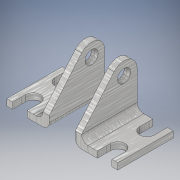
# Autodesk Inventor part: CylinderPivotMount_1.0625
Saved by Autodesk Inventor 2017 (Build 210142000, 142)
## iProperties
Created: 2017-01-24
Part Number: CylinderPivotMount_1.0625
Material: Steel
Document SubType Name: Modeling
Designer: Beezy
Density: 7.85 g/cm^3
Appearance: Polished Brushed
Author: Beezy
Autodesk Inventor part; units mm, degrees
ref_plane "YZ Plane" through (0, 0, 0) normal (1, 0, 0) x (0, 1, 0)
ref_plane "XZ Plane" through (0, 0, 0) normal (0, 1, 0) x (-1, 0, 0)
ref_plane "XY Plane" through (0, 0, 0) normal (0, 0, 1) x (1, 0, 0)
sketch "Sketch1" plane through (0, 0, 0) normal (0, 0, 1) x (1, 0, 0)
  line L0 (0, 0) -> (0, 44.7575) construction
  line L1 (-26.924, 0) -> (-26.924, 3.048)
  line L2 (-26.924, 3.048) -> (-12.573, 3.048)
  line L3 (-9.398, 6.223) -> (-9.398, 26.924)
  line L4 (-9.398, 26.924) -> (-6.35, 26.924)
  line L5 (-6.35, 26.924) -> (-6.35, 3.175)
  line L6 (-9.525, 0) -> (-26.924, 0)
  arc A0 (-9.525, 0) -> (-6.35, 3.175) centre (-9.525, 3.175) ccw
  arc A1 (-12.573, 3.048) -> (-9.398, 6.223) centre (-12.573, 6.223) ccw
  line L7 (26.924, 0) -> (26.924, 3.048)
  line L8 (26.924, 3.048) -> (12.573, 3.048)
  line L9 (9.398, 6.223) -> (9.398, 26.924)
  line L10 (9.398, 26.924) -> (6.35, 26.924)
  line L11 (6.35, 26.924) -> (6.35, 3.175)
  line L12 (9.525, 0) -> (26.924, 0)
  arc A2 (6.35, 3.175) -> (9.525, 0) centre (9.525, 3.175) ccw
  arc A3 (9.398, 6.223) -> (12.573, 3.048) centre (12.573, 6.223) ccw
  point P0 (-6.35, 0)
  point P1 (6.35, 0)
  dimension "d0" = 3.048
  dimension "d1" = 26.924
  dimension "d2" = 26.924
  dimension "d3" = 6.35
  dimension "d4" = 3.175
  constraints: 26 end point, 11 symmetric about line, 8 point on circle, 6 perpendicular, 4 centre point, 4 point on line, 4 tangent, 2 vertical, 1 equal radius, 1 horizontal alignment, 2 other
  measures "d0" distance of L1.start L1.end
  measures "d1" distance between parallel lines of L0 L1
  measures "d2" distance between parallel lines of L4 L6
  measures "d3" distance between parallel lines of L0 L5
  measures "d4" radius of A0
extrude "Extrusion1" add sketch "Sketch1" against normal blind 26.924
sketch "Sketch2" plane through (26.924, 0, 0) normal (1, 0, 0) x (0, 0, -1)
  line L0 (0, 6.223) -> (0, 26.924) projected
  line L1 (0, 6.223) -> (26.924, 6.223) projected
  line L2 (26.924, 26.924) -> (26.924, 6.223) projected
  line L3 (0, 26.924) -> (26.924, 26.924) projected
  line L4 (0, 3.048) -> (0, 6.223) projected
  line L5 (0, 3.048) -> (26.924, 3.048) projected
  line L6 (26.924, 6.223) -> (26.924, 3.048) projected
  line L7 (0, 6.223) -> (26.924, 6.223) projected
  line L8 (0, 0) -> (0, 3.048) projected
  line L9 (0, 0) -> (26.924, 0) projected
  line L10 (26.924, 3.048) -> (26.924, 0) projected
  line L11 (0, 3.048) -> (26.924, 3.048) projected
  circle A0 centre (20.574, 20.574) radius 3.175
  line L12 (26.924, 26.924) -> (26.924, 3.175) projected
  arc A1 (20.574, 26.924) -> (15.7411, 24.6929) centre (20.574, 20.574) ccw
  line L13 (15.7411, 24.6929) -> (0, 6.223)
  line L14 (0, 6.223) -> (26.924, 6.223) projected
  line L15 (0, 26.924) -> (26.924, 26.924) projected
  line L16 (20.574, 26.924) -> (0, 26.924)
  line L17 (0, 26.924) -> (0, 6.223)
  point P0 (0, 0)
  dimension "d7" = 6.35
  dimension "d8" = 6.35
  dimension "d9" = 6.35
  dimension "d10" = 6.35
  constraints: 6 end point, 2 centre point, 2 point on circle, 1 coincident, 1 tangent, 1 vertical alignment
  measures "d7" diameter of A0
  measures "d8" distance from line of L2 A0.centre
  measures "d9" distance from line of L3 A0.centre
  measures "d10" radius of A1
extrude "Extrusion2" cut sketch "Sketch2" against normal through all contours L0 L3 A1 L13 | A0
fillet "Fillet1" radius 6.35 2 edges at (7.874, 26.924, -26.924) (-7.874, 26.924, -26.924)
sketch "Sketch3" plane through (-26.924, 3.048, 0) normal (0, 1, 0) x (1, 0, 0)
  line L0 (0, 0) -> (14.351, 0) projected
  line L1 (14.351, 0) -> (14.351, 26.924) projected
  line L2 (0, 26.924) -> (14.351, 26.924) projected
  line L3 (0, 0) -> (0, 26.924) projected
  line L4 (53.848, 0) -> (39.497, 0) projected
  line L5 (53.848, 0) -> (53.848, 26.924) projected
  line L6 (39.497, 26.924) -> (53.848, 26.924) projected
  line L7 (39.497, 0) -> (39.497, 26.924) projected
  arc A0 (9.906, 6.35) -> (2.794, 6.35) centre (6.35, 6.35) ccw
  line L8 (9.906, 6.35) -> (9.906, 0)
  line L9 (2.794, 6.35) -> (2.794, 0)
  line L10 (17.399, 0) -> (0, 0) projected
  line L11 (0, 0) -> (0, 26.924) projected
  line L12 (0, 13.462) -> (53.848, 13.462) construction
  line L13 (26.924, 0) -> (26.924, 26.924) construction
  line L14 (2.794, 0) -> (9.906, 0)
  arc A1 (2.794, 20.574) -> (9.906, 20.574) centre (6.35, 20.574) ccw
  line L15 (9.906, 20.574) -> (9.906, 26.924)
  line L16 (2.794, 20.574) -> (2.794, 26.924)
  line L17 (2.794, 26.924) -> (9.906, 26.924)
  arc A2 (51.054, 6.35) -> (43.942, 6.35) centre (47.498, 6.35) ccw
  line L18 (43.942, 6.35) -> (43.942, 0)
  line L19 (51.054, 6.35) -> (51.054, 0)
  line L20 (51.054, 0) -> (43.942, 0)
  line L21 (43.942, 20.574) -> (43.942, 26.924)
  line L22 (51.054, 26.924) -> (43.942, 26.924)
  line L23 (51.054, 20.574) -> (51.054, 26.924)
  arc A3 (43.942, 20.574) -> (51.054, 20.574) centre (47.498, 20.574) ccw
  dimension "d14" = 6.35
  dimension "d15" = 7.112
  dimension "d16" = 6.35
  constraints: 28 end point, 15 symmetric about line, 8 point on circle, 4 centre point, 3 vertical, 2 midpoint, 2 point on line, 2 tangent, 1 collinear, 3 other
  measures "d14" distance from line of L0 A0.centre
  measures "d15" distance between parallel lines of L8 L9
  measures "d16" distance from line of L3 A0.centre
extrude "Extrusion3" cut sketch "Sketch3" against normal through all contours L9 A0 L8 L0 | L2 L15 A1 L16 | L4 L18 A2 L19 | L23 A3 L21 L6
body "Solid1"
